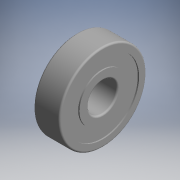
# Autodesk Inventor part: bearing_6200
Saved by Autodesk Inventor 2017.3 (Build 213256000, 256)
## iProperties
Part Number: bearing_6200
Material: Generic
Catalog Web Link: www.cadenas.de
Description: 6000_bearing-Deep Groove Ball Bearings
Vendor: MISUMI
Document SubType Name: Modeling
Designer: partserver
Manufacturer: MISUMI
Mass: 5.39446 g
Surface Area: 24.3498 cm^2
Volume: 5.39446 cm^3
Density: 1 g/cm^3
Appearance: PSOLRGB-192-192-192
Category: PARTsolutions
Company: MISUMI
Title: bearing_6200
Author: Cadenas PARTsolutions
Comments: Deep Groove Ball Bearings
PSOL_IDENT_0: {$CADENAS_DATA\23d-libs\misumi\metric\accessories\bearing_6000.prj},170 {VTYP=3D},{NB=bearing_6200},
PSOL_IDENT_1: {LINA=bearing_6200},{NN=6000_bearing},{DATE=30.10.2020 15:47:11},{GEOMDATE=24.10.2013 00:00:00},{VER
PSOL_IDENT_2: SION=},{LINEID=50},{WBVAR=},{WBNUMERIC=}  {NB=bearing_6200},{LINA=bearing_6200},{KT=DUMMY},{PN=beari
PSOL_IDENT_3: ng_6200},{BN=6200},{DD=10},{D=30},{B=9},{RR=0.6},{DSMIN=14.0},{DS1=16.00},{DSMAX=16.00},{DDHH=26.0},
PSOL_IDENT_4: {R=0.6},{R1=0.400},{R2=0.500},{MASS=32},{MASS11=32},{AA=8.1340},{BB=2.5500},{CC=3.1500},{DD1=28.170}
NB: bearing_6200
NN: 6000_bearing
NT: Deep Groove Ball Bearings
NBSYN: $PN.
LINA: bearing_6200
CATALOG: Misumi
PN: bearing_6200
BN: 6200
DD: 10
D: 30
B: 9
RR: 0.6
DSMIN: 14
DDHH: 26
R: 0.6
MASS11: 32
SUPPLIER: MISUMI
ARTICLENO: bearing_6200
BOMINFO: bearing_6200
CREATOR: CADENAS GmbH
Autodesk Inventor part; units mm, degrees
sketch "Sketch_1" plane through (0, 0, 0) normal (0, 0, 1) x (1, 0, 0)
  line L0 (9, 0) -> (0, 0)
  arc A0 (0, 5.6) -> (0.6, 5) centre (0.6, 5.6) ccw
  line L1 (0.6, 5) -> (8.4, 5)
  arc A1 (8.4, 5) -> (9, 5.6) centre (8.4, 5.6) ccw
  line L2 (9, 5.6) -> (9, 8.15)
  line L3 (9, 8.15) -> (8.567, 8.15)
  line L4 (8.567, 8.15) -> (8.567, 12.45)
  line L5 (8.567, 12.45) -> (9, 12.45)
  line L6 (9, 12.45) -> (9, 14.4)
  arc A2 (9, 14.4) -> (8.4, 15) centre (8.4, 14.4) ccw
  line L7 (8.4, 15) -> (0.6, 15)
  arc A3 (0.6, 15) -> (0, 14.4) centre (0.6, 14.4) ccw
  line L8 (0, 14.4) -> (0, 12.45)
  line L9 (0, 12.45) -> (0.433, 12.45)
  line L10 (0.433, 12.45) -> (0.433, 8.15)
  line L11 (0.433, 8.15) -> (0, 8.15)
  line L12 (0, 8.15) -> (0, 5.6)
  constraints: 26 end point, 8 point on circle, 4 centre point
revolve "Revolution1" add sketch "Sketch_1" angle 360 about axis through (9, 0, 0) along (1, 0, 0)
ref_plane "center_point_XY" through (4.5, 0, 0) normal (1, 0, 0) x (0, 0, -1)
ref_plane "center_point_YZ" through (4.5, 0, 0) normal (0, 0, -1) x (0, 1, 0)
ref_plane "center_point_ZX" through (4.5, 0, 0) normal (0, 1, 0) x (1, 0, 0)
ref_plane "to_housing_XY" through (0, 0, 0) normal (1, 0, 0) x (0, 0, -1)
ref_plane "to_housing_YZ" through (0, 0, 0) normal (0, 0, -1) x (0, 1, 0)
ref_plane "to_housing_ZX" through (0, 0, 0) normal (0, 1, 0) x (1, 0, 0)
ref_plane "to_ring_XY" through (8.134, 0, 0) normal (1, 0, 0) x (0, 0, -1)
ref_plane "to_ring_YZ" through (8.134, 0, 0) normal (0, 0, -1) x (0, 1, 0)
ref_plane "to_ring_ZX" through (8.134, 0, 0) normal (0, 1, 0) x (1, 0, 0)
body "Solid1"
